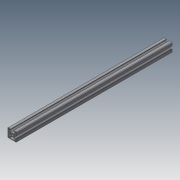
# Autodesk Inventor part: Standard
Saved by Autodesk Inventor 2020.3 (Build 243373000, 373)
## iProperties
RuleStatus: InUse
AfterDocSave0: file://Part Number Cleaner
Created: 2023-03-27
Material: Generic
Catalog Web Link: https://www.janelia.org/
Vendor: HHMI: JRC - jET
Document SubType Name: Modeling
Designer: arnoldj
Density: 1 g/cm^3
Appearance: Default
DESIGN DEPARTMENT: HHMI: JRC - jET
ALTERED ITEM PART NUMBER: N/A
ALTERED ITEM VENDOR: N/A
ALTERED ITEM DESCRIPTION: N/A
Title: Standard
Author: arnoldj
Revision Number: 0
Autodesk Inventor part; units mm, degrees
ref_plane "YZ Plane" through (0, 0, 0) normal (1, 0, 0) x (0, 1, 0)
ref_plane "XZ Plane" through (0, 0, 0) normal (0, 1, 0) x (-1, 0, 0)
ref_plane "XY Plane" through (0, 0, 0) normal (0, 0, 1) x (1, 0, 0)
feature "Boss-Extrude1" [suppressed]
sketch "Sketch1" plane through (0, 0, 0) normal (0, 0, 1) x (1, 0, 0)
  arc A0 (-15, -13) -> (-13, -15) centre (-13, -13) ccw projected
  line L0 (-13, -15) -> (13, -15) projected
  arc A1 (13, -15) -> (15, -13) centre (13, -13) ccw projected
  line L1 (15, -13) -> (15, -4.75) projected
  arc A2 (15, -4.75) -> (14.8, -4.55) centre (14.8, -4.75) ccw projected
  line L2 (14.8, -4.55) -> (14.7, -4.55) projected
  arc A3 (14.5, -4.35) -> (14.7, -4.55) centre (14.7, -4.35) ccw projected
  line L3 (14.5, -4.35) -> (14.5, -4.25) projected
  arc A4 (14.5, -4.25) -> (14.3, -4.05) centre (14.3, -4.25) ccw projected
  line L4 (14.3, -4.05) -> (13.4, -4.05) projected
  arc A5 (13.4, -4.05) -> (12.8, -4.65) centre (13.4, -4.65) ccw projected
  line L5 (12.8, -4.65) -> (12.8, -8.05) projected
  arc A6 (12.6, -8.25) -> (12.8, -8.05) centre (12.6, -8.05) ccw projected
  line L6 (12.6, -8.25) -> (10.05, -8.25) projected
  line L7 (10.05, -8.25) -> (6.0044, -4.2045) projected
  line L8 (6.0044, -4.2045) -> (6.0044, 4.2045) projected
  line L9 (6.0044, 4.2045) -> (10.05, 8.25) projected
  line L10 (10.05, 8.25) -> (12.6, 8.25) projected
  arc A7 (12.8, 8.05) -> (12.6, 8.25) centre (12.6, 8.05) ccw projected
  line L11 (12.8, 8.05) -> (12.8, 4.65) projected
  arc A8 (12.8, 4.65) -> (13.4, 4.05) centre (13.4, 4.65) ccw projected
  line L12 (13.4, 4.05) -> (14.3, 4.05) projected
  arc A9 (14.3, 4.05) -> (14.5, 4.25) centre (14.3, 4.25) ccw projected
  line L13 (14.5, 4.25) -> (14.5, 4.35) projected
  arc A10 (14.7, 4.55) -> (14.5, 4.35) centre (14.7, 4.35) ccw projected
  line L14 (14.7, 4.55) -> (14.8, 4.55) projected
  arc A11 (14.8, 4.55) -> (15, 4.75) centre (14.8, 4.75) ccw projected
  line L15 (15, 4.75) -> (15, 13) projected
  arc A12 (15, 13) -> (13, 15) centre (13, 13) ccw projected
  line L16 (13, 15) -> (4.75, 15) projected
  arc A13 (4.75, 15) -> (4.55, 14.8) centre (4.75, 14.8) ccw projected
  line L17 (4.55, 14.8) -> (4.55, 14.7) projected
  arc A14 (4.35, 14.5) -> (4.55, 14.7) centre (4.35, 14.7) ccw projected
  line L18 (4.35, 14.5) -> (4.25, 14.5) projected
  arc A15 (4.25, 14.5) -> (4.05, 14.3) centre (4.25, 14.3) ccw projected
  line L19 (4.05, 14.3) -> (4.05, 13.4) projected
  arc A16 (4.05, 13.4) -> (4.65, 12.8) centre (4.65, 13.4) ccw projected
  line L20 (4.65, 12.8) -> (8.05, 12.8) projected
  arc A17 (8.25, 12.6) -> (8.05, 12.8) centre (8.05, 12.6) ccw projected
  line L21 (8.25, 12.6) -> (8.25, 10.05) projected
  line L22 (8.25, 10.05) -> (4.2045, 6.0044) projected
  line L23 (4.2045, 6.0044) -> (-4.2045, 6.0044) projected
  line L24 (-4.2045, 6.0044) -> (-8.25, 10.05) projected
  line L25 (-8.25, 10.05) -> (-8.25, 12.6) projected
  arc A18 (-8.05, 12.8) -> (-8.25, 12.6) centre (-8.05, 12.6) ccw projected
  line L26 (-8.05, 12.8) -> (-4.65, 12.8) projected
  arc A19 (-4.65, 12.8) -> (-4.05, 13.4) centre (-4.65, 13.4) ccw projected
  line L27 (-4.05, 13.4) -> (-4.05, 14.3) projected
  arc A20 (-4.05, 14.3) -> (-4.25, 14.5) centre (-4.25, 14.3) ccw projected
  line L28 (-4.25, 14.5) -> (-4.35, 14.5) projected
  arc A21 (-4.55, 14.7) -> (-4.35, 14.5) centre (-4.35, 14.7) ccw projected
  line L29 (-4.55, 14.7) -> (-4.55, 14.8) projected
  arc A22 (-4.55, 14.8) -> (-4.75, 15) centre (-4.75, 14.8) ccw projected
  line L30 (-4.75, 15) -> (-13, 15) projected
  arc A23 (-13, 15) -> (-15, 13) centre (-13, 13) ccw projected
  line L31 (-15, 13) -> (-15, -13) projected
  circle A24 centre (0, 0) radius 3.5 projected
  arc A25 (12.7, -13.7) -> (13.7, -12.7) centre (12.7, -12.7) ccw projected
  line L32 (10.5, -13.7) -> (12.7, -13.7) projected
  arc A26 (9.5, -12.7) -> (10.5, -13.7) centre (10.5, -12.7) ccw projected
  line L33 (9.5, -10.5) -> (9.5, -12.7) projected
  arc A27 (10.5, -9.5) -> (9.5, -10.5) centre (10.5, -10.5) ccw projected
  line L34 (12.7, -9.5) -> (10.5, -9.5) projected
  arc A28 (13.7, -10.5) -> (12.7, -9.5) centre (12.7, -10.5) ccw projected
  line L35 (13.7, -12.7) -> (13.7, -10.5) projected
  arc A29 (13.7, 12.7) -> (12.7, 13.7) centre (12.7, 12.7) ccw projected
  line L36 (13.7, 10.5) -> (13.7, 12.7) projected
  arc A30 (12.7, 9.5) -> (13.7, 10.5) centre (12.7, 10.5) ccw projected
  line L37 (10.5, 9.5) -> (12.7, 9.5) projected
  arc A31 (9.5, 10.5) -> (10.5, 9.5) centre (10.5, 10.5) ccw projected
  line L38 (9.5, 12.7) -> (9.5, 10.5) projected
  arc A32 (10.5, 13.7) -> (9.5, 12.7) centre (10.5, 12.7) ccw projected
  line L39 (12.7, 13.7) -> (10.5, 13.7) projected
  arc A33 (8.05, -12.8) -> (8.25, -12.6) centre (8.05, -12.6) ccw projected
  line L40 (-8.05, -12.8) -> (8.05, -12.8) projected
  arc A34 (-8.25, -12.6) -> (-8.05, -12.8) centre (-8.05, -12.6) ccw projected
  line L41 (-8.25, -10.05) -> (-8.25, -12.6) projected
  line L42 (-4.2045, -6.0044) -> (-8.25, -10.05) projected
  line L43 (4.2045, -6.0044) -> (-4.2045, -6.0044) projected
  line L44 (8.25, -10.05) -> (4.2045, -6.0044) projected
  line L45 (8.25, -12.6) -> (8.25, -10.05) projected
  arc A35 (-13.7, -12.7) -> (-12.7, -13.7) centre (-12.7, -12.7) ccw projected
  line L46 (-13.7, -10.5) -> (-13.7, -12.7) projected
  arc A36 (-12.7, -9.5) -> (-13.7, -10.5) centre (-12.7, -10.5) ccw projected
  line L47 (-10.5, -9.5) -> (-12.7, -9.5) projected
  arc A37 (-9.5, -10.5) -> (-10.5, -9.5) centre (-10.5, -10.5) ccw projected
  line L48 (-9.5, -12.7) -> (-9.5, -10.5) projected
  arc A38 (-10.5, -13.7) -> (-9.5, -12.7) centre (-10.5, -12.7) ccw projected
  line L49 (-12.7, -13.7) -> (-10.5, -13.7) projected
  arc A39 (-12.7, 13.7) -> (-13.7, 12.7) centre (-12.7, 12.7) ccw projected
  line L50 (-10.5, 13.7) -> (-12.7, 13.7) projected
  arc A40 (-9.5, 12.7) -> (-10.5, 13.7) centre (-10.5, 12.7) ccw projected
  line L51 (-9.5, 10.5) -> (-9.5, 12.7) projected
  arc A41 (-10.5, 9.5) -> (-9.5, 10.5) centre (-10.5, 10.5) ccw projected
  line L52 (-12.7, 9.5) -> (-10.5, 9.5) projected
  arc A42 (-13.7, 10.5) -> (-12.7, 9.5) centre (-12.7, 10.5) ccw projected
  line L53 (-13.7, 12.7) -> (-13.7, 10.5) projected
  arc A43 (-12.8, -8.05) -> (-12.6, -8.25) centre (-12.6, -8.05) ccw projected
  line L54 (-12.8, 8.05) -> (-12.8, -8.05) projected
  arc A44 (-12.6, 8.25) -> (-12.8, 8.05) centre (-12.6, 8.05) ccw projected
  line L55 (-10.05, 8.25) -> (-12.6, 8.25) projected
  line L56 (-6.0044, 4.2045) -> (-10.05, 8.25) projected
  line L57 (-6.0044, -4.2045) -> (-6.0044, 4.2045) projected
  line L58 (-10.05, -8.25) -> (-6.0044, -4.2045) projected
  line L59 (-12.6, -8.25) -> (-10.05, -8.25) projected
  point P0 (0, 0)
extrude "Extrusion1" add sketch "Sketch1" along normal mid plane 524
body "Solid1"
